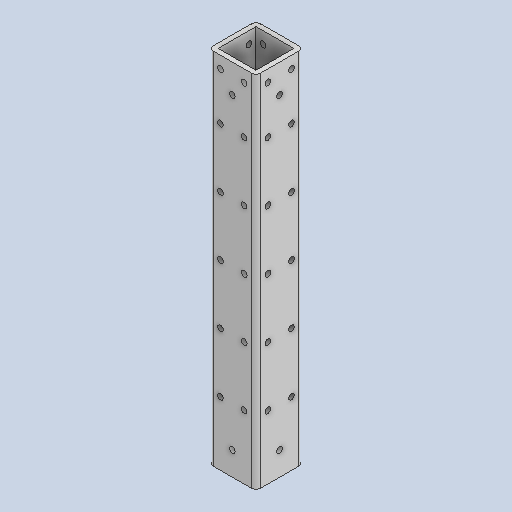
# Autodesk Inventor part: verticalaxle
Saved by Autodesk Inventor 2025.4 (Build 294407000, 407)
## iProperties
Created: 2026-03-22
Part Number: verticalaxle
Material: Generic
Document SubType Name: Modeling
Designer: hp
Density: 1 g/cm^3
Appearance: Default
Author: hp
Autodesk Inventor part; units mm, degrees
ref_plane "YZ Plane" through (0, 0, 0) normal (1, 0, 0) x (0, 1, 0)
ref_plane "XZ Plane" through (0, 0, 0) normal (0, 1, 0) x (-1, 0, 0)
ref_plane "XY Plane" through (0, 0, 0) normal (0, 0, 1) x (1, 0, 0)
sketch "Sketch1" plane through (0, 0, 0) normal (0, 1, 0) x (-1, 0, 0)
  line L0 (8, 10) -> (-8, 10)
  line L1 (-10, 8) -> (-10, -8)
  line L2 (-8, -10) -> (8, -10)
  line L3 (10, -8) -> (10, 8)
  line L4 (10, 10) -> (-10, -10) construction
  line L5 (-10, 10) -> (10, -10) construction
  line L6 (8, 8) -> (-8, 8)
  line L7 (-8, 8) -> (-8, -8)
  line L8 (-8, -8) -> (8, -8)
  line L9 (8, -8) -> (8, 8)
  arc A0 (10, 8) -> (8, 10) centre (8, 8) ccw
  arc A1 (8, -10) -> (10, -8) centre (8, -8) ccw
  arc A2 (-10, -8) -> (-8, -10) centre (-8, -8) ccw
  arc A3 (-8, 10) -> (-10, 8) centre (-8, 8) ccw
  point P0 (0, 0)
  dimension "d0" = 20
  dimension "d1" = 20
  dimension "d2" = 2
  dimension "d3" = 2
  constraints: 20 end point, 8 point on circle, 8 point on line, 8 tangent, 4 centre point, 4 parallel, 3 equal radius, 2 midpoint, 2 perpendicular, 1 horizontal, 3 other
  measures "d0" distance of L5.end L4.end
  measures "d1" distance of L4.end L5.start
  measures "d2" distance between parallel lines of L3 L9
  measures "d3" radius of A0
extrude "Extrusion1" add sketch "Sketch1" along normal blind 152
sketch "Sketch2" plane through (10, 0, 8) normal (1, 0, 0) x (0, 0, -1)
  line L0 (0, 0) -> (0, 152) projected
  line L1 (16, 0) -> (16, 152) projected
  line L2 (0, 0) -> (16, 0) projected
  line L3 (0, 152) -> (16, 152) projected
  line L4 (8, 29.2747) -> (8, 0) construction
  line L5 (8, 127) -> (8, 177) construction
  line L6 (8, 102) -> (8, 202) construction
  line L7 (8, 77) -> (8, 227) construction
  line L8 (8, 52) -> (8, 252) construction
  point P0 (8, 0)
  point P1 (8, 140)
  point P2 (8, 10)
  point P3 (3, 127)
  point P4 (3, 102)
  point P5 (3, 77)
  point P6 (3, 52)
  point P7 (3, 27)
  point P8 (13, 127)
  point P9 (13, 102)
  point P10 (13, 77)
  point P11 (13, 52)
  point P12 (13, 27)
  point P13 (3, 147)
  point P14 (13, 147)
  point P15 (8, 76)
  dimension "d6" = 140
  dimension "d7" = 8
  dimension "d22" = 142
  dimension "d23" = 5
  dimension "d24" = 127
  dimension "d27" = 127
  dimension "d130" = 10
  dimension "d159" = 147
  dimension "d160" = 76
  constraints: 10 end point, 5 symmetric about line, 1 point on line, 1 vertical, 7 other
  measures "d6" distance from line of L2 point (8, 140)
  measures "d7" distance from line of point (8, 140) L0
  measures "d22" distance from line of point (8, 10) L3
  measures "d23" distance from line of L4 point (3, 127)
  measures "d24" distance from line of L2 point (3, 127)
  measures "d27" distance of point (8, 0) L5.start
  measures "d130" distance of point (13, 147) point (3, 147)
  measures "d159" distance from line of L2 point (3, 147)
  measures "d160" distance from line of L2 point (8, 76)
hole "Hole1" at (10, 140, 0) at (10, 10, 0) direction (-1, 0, 0) diameter 2.45 depth 2
pattern_circular "Circular Pattern1" count 4 over 360 about axis through (0, -10, 0) along (0, 1, 0) of "Hole1"
thread "Thread1" size "M2.5x0.45" class "6H" standard "ANSI Metric M Profile" full length
thread "Thread2" size "M2.5x0.45" class "6H" standard "ANSI Metric M Profile" full length
hole "Hole2" at (10, 27, 5) at (10, 27, -5) at (10, 52, -5) at (10, 52, 5) at (10, 77, -5) at (10, 77, 5) at (10, 102, 5) at (10, 102, -5) at (10, 127, 5) at (10, 127, -5) direction (-1, 0, 0) diameter 2.45 depth 2
thread "Thread3" size "M2.5x0.45" class "6H" standard "ISO Metric profile" length 8
thread "Thread4" size "M2.5x0.45" class "6H" standard "ISO Metric profile" length 8
thread "Thread5" size "M2.5x0.45" class "6H" standard "ISO Metric profile" length 8
thread "Thread6" size "M2.5x0.45" class "6H" standard "ISO Metric profile" length 8
thread "Thread7" size "M2.5x0.45" class "6H" standard "ISO Metric profile" length 8
thread "Thread8" size "M2.5x0.45" class "6H" standard "ISO Metric profile" length 8
thread "Thread9" size "M2.5x0.45" class "6H" standard "ISO Metric profile" length 8
thread "Thread10" size "M2.5x0.45" class "6H" standard "ISO Metric profile" length 8
thread "Thread11" size "M2.5x0.45" class "6H" standard "ISO Metric profile" length 8
thread "Thread12" size "M2.5x0.45" class "6H" standard "ISO Metric profile" length 8
thread "Thread13" size "M2.5x0.45" class "6H" standard "ISO Metric profile" length 8
pattern_circular "Circular Pattern2" count 4 over 360 about axis through (0, -10, 0) along (0, 1, 0) of "Hole2"
thread "Thread14" size "M2.5x0.45" class "6H" standard "ISO Metric profile" length 8
thread "Thread15" size "M2.5x0.45" class "6H" standard "ISO Metric profile" length 8
thread "Thread16" size "M2.5x0.45" class "6H" standard "ISO Metric profile" length 8
thread "Thread17" size "M2.5x0.45" class "6H" standard "ISO Metric profile" length 8
thread "Thread18" size "M2.5x0.45" class "6H" standard "ISO Metric profile" length 8
thread "Thread19" size "M2.5x0.45" class "6H" standard "ISO Metric profile" length 8
thread "Thread20" size "M2.5x0.45" class "6H" standard "ISO Metric profile" length 8
thread "Thread21" size "M2.5x0.45" class "6H" standard "ISO Metric profile" length 8
thread "Thread22" size "M2.5x0.45" class "6H" standard "ISO Metric profile" length 8
thread "Thread23" size "M2.5x0.45" class "6H" standard "ISO Metric profile" length 8
thread "Thread24" size "M2.5x0.45" class "6H" standard "ISO Metric profile" length 8
thread "Thread25" size "M2.5x0.45" class "6H" standard "ISO Metric profile" length 8
thread "Thread26" size "M2.5x0.45" class "6H" standard "ISO Metric profile" length 8
thread "Thread27" size "M2.5x0.45" class "6H" standard "ISO Metric profile" length 8
thread "Thread28" size "M2.5x0.45" class "6H" standard "ISO Metric profile" length 8
thread "Thread29" size "M2.5x0.45" class "6H" standard "ISO Metric profile" length 8
thread "Thread30" size "M2.5x0.45" class "6H" standard "ISO Metric profile" length 8
thread "Thread31" size "M2.5x0.45" class "6H" standard "ISO Metric profile" length 8
thread "Thread32" size "M2.5x0.45" class "6H" standard "ISO Metric profile" length 8
thread "Thread33" size "M2.5x0.45" class "6H" standard "ISO Metric profile" length 8
thread "Thread34" size "M2.5x0.45" class "6H" standard "ISO Metric profile" length 8
thread "Thread35" size "M2.5x0.45" class "6H" standard "ISO Metric profile" length 8
thread "Thread36" size "M2.5x0.45" class "6H" standard "ISO Metric profile" length 8
thread "Thread37" size "M2.5x0.45" class "6H" standard "ISO Metric profile" length 8
thread "Thread38" size "M2.5x0.45" class "6H" standard "ISO Metric profile" length 8
thread "Thread39" size "M2.5x0.45" class "6H" standard "ISO Metric profile" length 8
thread "Thread40" size "M2.5x0.45" class "6H" standard "ISO Metric profile" length 8
thread "Thread41" size "M2.5x0.45" class "6H" standard "ISO Metric profile" length 8
thread "Thread42" size "M2.5x0.45" class "6H" standard "ISO Metric profile" length 8
thread "Thread43" size "M2.5x0.45" class "6H" standard "ISO Metric profile" length 8
thread "Thread44" size "M2.5x0.45" class "6H" standard "ISO Metric profile" length 8
thread "Thread45" size "M2.5x0.45" class "6H" standard "ISO Metric profile" length 8
thread "Thread46" size "M2.5x0.45" class "6H" standard "ISO Metric profile" length 8
hole "Hole3" at (10, 147, 5) at (10, 147, -5) direction (-1, 0, 0) diameter 2.45 depth 2
thread "Thread47" size "M2.5x0.45" class "6H" standard "ISO Metric profile" length 8
thread "Thread48" size "M2.5x0.45" class "6H" standard "ISO Metric profile" length 8
pattern_circular "Circular Pattern3" count 4 over 360 about axis through (0, -10, 0) along (0, 1, 0) of "Hole3"
thread "Thread49" size "M2.5x0.45" class "6H" standard "ISO Metric profile" length 8
thread "Thread50" size "M2.5x0.45" class "6H" standard "ISO Metric profile" length 8
thread "Thread51" size "M2.5x0.45" class "6H" standard "ISO Metric profile" length 9.967
thread "Thread52" size "M2.5x0.45" class "6H" standard "ISO Metric profile" length 9.967
thread "Thread53" size "M2.5x0.45" class "6H" standard "ISO Metric profile" length 9.967
thread "Thread54" size "M2.5x0.45" class "6H" standard "ISO Metric profile" length 9.967
body "Solid1"
